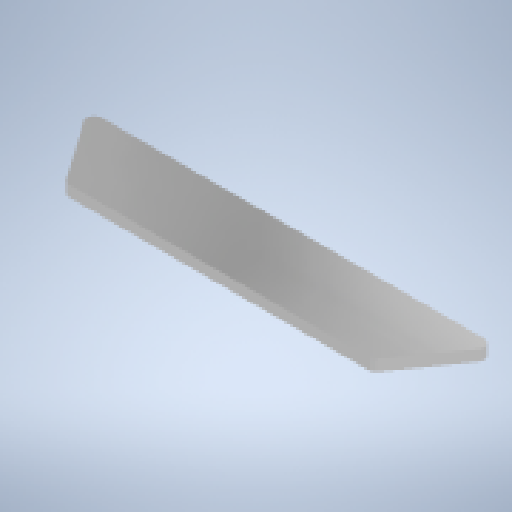
# Autodesk Inventor part: shield_side_side
Saved by Autodesk Inventor 2024.1 (Build 281209000, 209)
## iProperties
Created: 2024-02-14
Part Number: shield_side_side
Material: アルミニウム 6061
Document SubType Name: Modeling
Designer: hibik
Density: 2.7 g/cm^3
Appearance: アルミニウム - フラット
Author: hibik
Autodesk Inventor part; units mm, degrees
ref_plane "YZ Plane" through (0, 0, 0) normal (1, 0, 0) x (0, 1, 0)
ref_plane "XZ Plane" through (0, 0, 0) normal (0, 1, 0) x (-1, 0, 0)
ref_plane "XY Plane" through (0, 0, 0) normal (0, 0, 1) x (1, 0, 0)
sketch "スケッチ1" plane through (0, 0, 0) normal (0, 1, 0) x (-1, 0, 0)
  line L0 (55, 0) -> (0, 0)
  line L1 (0, 0) -> (0, -20)
  line L2 (0, -20) -> (55, -20)
  line L3 (55, -20) -> (55, 0)
  dimension "d0" = 20
  dimension "d1" = 55
  constraints: 8 end point, 2 parallel, 1 coincident, 1 horizontal, 1 perpendicular
  measures "d0" distance of L0.end L1.end
  measures "d1" distance of L0.start L0.end
extrude "押し出し1" add sketch "スケッチ1" along normal blind 1.5
sketch "スケッチ2" plane through (0, 0, 0) normal (0, -1, 0) x (1, 0, 0)
  line L0 (-7, -10.1005) -> (0, -20) projected
  line L1 (-7, -10.1005) -> (-48, -10.1005) projected
  line L2 (0, -20) -> (-55, -20) projected
  line L3 (-48, -10.1005) -> (-55, -20) projected
  line L4 (0, 0) -> (0, -20) projected
  line L5 (-55, 0) -> (0, 0) projected
  line L6 (-55, -20) -> (-55, 0) projected
  line L7 (0, -20) -> (-55, -20) projected
  point P0 (0, -20)
extrude "押し出し2" cut sketch "スケッチ2" against normal through all contours L1 L3 L6 L5 L4 L0
fillet "フィレット1" radius 1 4 edges at (-7, 0.75, -10.1005) (0, 0.75, -20) (-48, 0.75, -10.1005) (-55, 0.75, -20)
